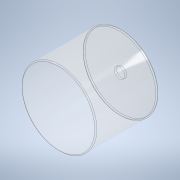
# Autodesk Inventor part: expo7
Saved by Autodesk Inventor 2020 (Build 240168000, 168)
## iProperties
Created: 2020-03-01
Part Number: expo7
Material: Glass, Cast, Clear
Document SubType Name: Modeling
Designer: Aryan
Density: 2.18 g/cm^3
Appearance: Clear
Author: Aryan
Autodesk Inventor part; units mm, degrees
ref_plane "YZ Plane" through (0, 0, 0) normal (1, 0, 0) x (0, 1, 0)
ref_plane "XZ Plane" through (0, 0, 0) normal (0, 1, 0) x (-1, 0, 0)
ref_plane "XY Plane" through (0, 0, 0) normal (0, 0, 1) x (1, 0, 0)
sketch "Sketch7" plane through (0, 0, 0) normal (0, 0, 1) x (1, 0, 0)
  circle A0 centre (0, 0) radius 35.5
  dimension "d32" = 71
  constraints: 1 centre point, 1 coincident
  measures "d32" diameter of A0
extrude "Extrusion3" add sketch "Sketch7" along normal blind 60
sketch "Sketch9" plane through (0, 0, 60) normal (0, 0, 1) x (1, 0, 0)
  circle A0 centre (0, 0) radius 34.5
  dimension "d35" = 69
  constraints: 1 centre point, 1 coincident
  measures "d35" diameter of A0
extrude "Extrusion4" cut sketch "Sketch9" against normal blind 58
fillet "Fillet3" radius 1 1 edges at (-35.5, 0, 0)
fillet "Fillet4" radius 1 1 edges at (-35.5, 0, 60)
sketch "Sketch10" plane through (0, 0, 0) normal (0, 0, -1) x (-1, 0, 0)
  circle A0 centre (0, 0) radius 5
  dimension "d40" = 10
  constraints: 1 centre point, 1 coincident
  measures "d40" diameter of A0
hole "Hole4" at (0, 0, 0) direction (0, 0, 1) diameter 10 end through all
body "Solid2"
